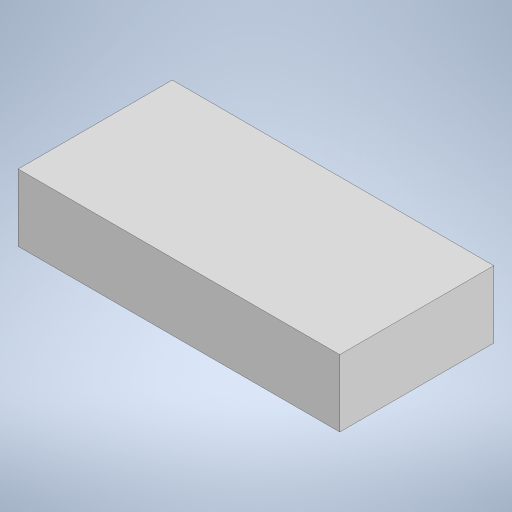
# Autodesk Inventor part: стабилизатор
Saved by Autodesk Inventor 2023.1 (Build 271208000, 208)
## iProperties
Created: 2025-01-21
Part Number: стабилизатор
Material: Типовые
Document SubType Name: Modeling
Designer: DELL
Density: 1 g/cm^3
Appearance: По умолчанию
Author: DELL
Autodesk Inventor part; units mm, degrees
ref_plane "YZ Plane" through (0, 0, 0) normal (1, 0, 0) x (0, 1, 0)
ref_plane "XZ Plane" through (0, 0, 0) normal (0, 1, 0) x (-1, 0, 0)
ref_plane "XY Plane" through (0, 0, 0) normal (0, 0, 1) x (1, 0, 0)
sketch "Эскиз1" plane through (0, 0, 0) normal (0, 1, 0) x (-1, 0, 0)
  line L0 (24, -11.5) -> (-24, -11.5)
  line L1 (-24, -11.5) -> (-24, 11.5)
  line L2 (-24, 11.5) -> (24, 11.5)
  line L3 (24, 11.5) -> (24, -11.5)
  line L4 (24, -11.5) -> (-24, 11.5) construction
  line L5 (-24, -11.5) -> (24, 11.5) construction
  point P0 (0, 0)
  dimension "d0" = 48
  dimension "d1" = 23
  constraints: 12 end point, 2 midpoint, 2 parallel, 1 horizontal, 1 perpendicular
  measures "d0" distance of L1.end L2.end
  measures "d1" distance of L0.end L1.end
extrude "Выдавливание1" add sketch "Эскиз1" along normal blind 10
